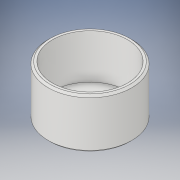
# Autodesk Inventor part: Flat Cap External 2 IN
Saved by Autodesk Inventor 2019 (Build 230136000, 136)
## iProperties
Created: 2019-07-06
Part Number: Flat Cap External 2 IN
Material: PVC-Piping
Document SubType Name: Modeling
Designer: J. LENDI
Mass: 53.5005 g
Surface Area: 218.475 cm^2
Volume: 38.2146 cm^3
Density: 1.4 g/cm^3
Appearance: Smooth - White
Author: J. LENDI
Autodesk Inventor part; units mm, degrees
ref_plane "YZ Plane" through (0, 0, 0) normal (1, 0, 0) x (0, 1, 0)
ref_plane "XZ Plane" through (0, 0, 0) normal (0, 1, 0) x (-1, 0, 0)
ref_plane "XY Plane" through (0, 0, 0) normal (0, 0, 1) x (1, 0, 0)
sketch "Sketch1" plane through (0, 0, 0) normal (0, 0, 1) x (1, 0, 0)
  line L0 (0, 19.9009) -> (0, -19.9009)
  line L1 (33.5661, 19.9009) -> (33.5661, -19.9009)
  line L2 (33.5661, -19.9009) -> (0, -19.9009)
  line L3 (33.5661, 19.9009) -> (30.1625, 19.9009)
  line L4 (30.1625, 19.9009) -> (30.1625, -15.8369)
  line L5 (30.1625, -15.8369) -> (0, -15.8369)
  point P0 (0, 0)
  dimension "d0" = 39.8018
  dimension "d1" = 19.9009
  dimension "d2" = 39.8018
  dimension "d3" = 19.9009
  dimension "d4" = 67.1322
  dimension "d5" = 60.325
  dimension "d7" = 35.7378
  constraints: 12 end point, 2 horizontal, 2 perpendicular, 2 vertical, 1 point on line
  measures "d0" distance of L0.start L0.end
  measures "d1" distance of point (0, 0) L0.start
  measures "d2" distance of L1.start L1.end
  measures "d3" vertical distance of point (0, 0) L1.start
  measures "d4" diameter of L1 L0
  measures "d5" diameter of L4 L0
  measures "d7" distance between parallel lines of L5 L3
revolve "Revolution1" add sketch "Sketch1" angle 360 about axis through (0, 19.9009, 0) along (0, -1, 0)
chamfer "Chamfer1" distance 1.5875 angle 45 2 edges at (-33.5661, 19.9009, 0) (-33.5661, -19.9009, 0)
equation "\"d0\" = d2"
equation "\"d1\" = 0.5 * d0"
equation "\"d3\" = 0.5 * d2"
body "Solid1"
